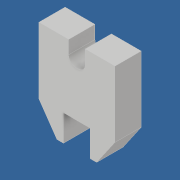
# Autodesk Inventor part: Base
Saved by Autodesk Inventor 2018 (Build 220112000, 112)
## iProperties
Created: 2017-12-20
Part Number: Base
Material: Generic
Document SubType Name: Modeling
Designer: 232963
Density: 1 g/cm^3
Appearance: Default
Author: 232963
Autodesk Inventor part; units mm, degrees
ref_plane "YZ Plane" through (0, 0, 0) normal (1, 0, 0) x (0, 1, 0)
ref_plane "XZ Plane" through (0, 0, 0) normal (0, 1, 0) x (-1, 0, 0)
ref_plane "XY Plane" through (0, 0, 0) normal (0, 0, 1) x (1, 0, 0)
sketch "Sketch1" plane through (0, 0, 0) normal (0, 0, 1) x (1, 0, 0)
  line L0 (73.279, 0) -> (73.279, 88.9)
  line L1 (0, 88.9) -> (0, 0)
  arc A0 (28.702, 76.2) -> (44.577, 76.2) centre (36.6395, 76.2) ccw
  line L2 (28.702, 76.2) -> (28.702, 88.9)
  line L3 (44.577, 76.2) -> (44.577, 88.9)
  line L4 (73.279, 88.9) -> (44.577, 88.9)
  line L5 (28.702, 88.9) -> (0, 88.9)
  line L6 (23.8252, 0) -> (49.4538, 0)
  line L7 (49.4538, 0) -> (49.4538, 25.4)
  line L8 (49.4538, 25.4) -> (23.8252, 25.4)
  line L9 (23.8252, 25.4) -> (23.8252, 0)
  line L10 (0, 25.4) -> (17.526, 0)
  line L11 (73.279, 25.4) -> (55.753, 0)
  line L12 (0, 0) -> (23.8252, 0)
  line L13 (49.4538, 0) -> (73.279, 0)
  dimension "d0" = 73.279
  dimension "d1" = 88.9
  dimension "d2" = 15.875
  dimension "d4" = 25.6286
  dimension "d5" = 63.5
  dimension "d6" = 23.8252
  dimension "d7" = 17.526
  dimension "d8" = 17.526
  constraints: 28 end point, 7 parallel, 7 perpendicular, 4 point on line, 3 horizontal, 2 point on circle, 2 tangent, 1 centre point
  measures "d0" distance of L1.start L0.end
  measures "d1" distance of L0.end L0.start
  measures "d2" diameter of A0
  measures "d4" distance of L8.end L7.end
  measures "d5" distance between parallel lines of L5 L8
  measures "d6" distance between parallel lines of L1 L9
  measures "d7" distance of L1.end L10.end
  measures "d8" distance of L0.start L11.end
extrude "Extrusion1" add sketch "Sketch1" along normal blind 25.4 contours L11 L13 L7 L8 L9 L12 L10 L1 L5 L2 A0 L3 L4 L0
body "Solid1"
